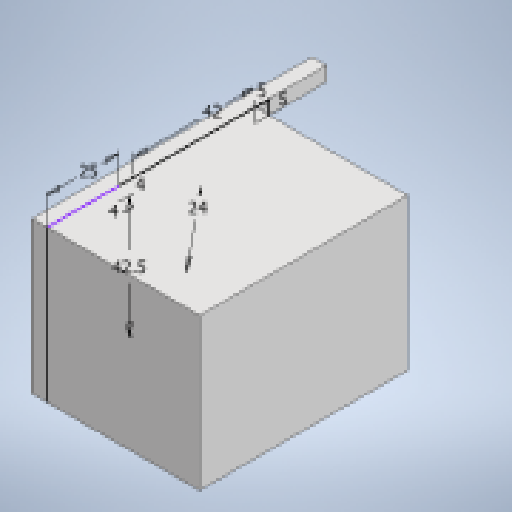
# Autodesk Inventor part: motor_mount
Saved by Autodesk Inventor 2023 (Build 270158000, 158)
## iProperties
Created: 2022-10-01
Part Number: motor_mount
Material: Generic
Document SubType Name: Modeling
Designer: carso
Density: 1 g/cm^3
Appearance: Default
Author: carso
Autodesk Inventor part; units mm, degrees
ref_plane "YZ Plane" through (0, 0, 0) normal (1, 0, 0) x (0, 1, 0)
ref_plane "XZ Plane" through (0, 0, 0) normal (0, 1, 0) x (-1, 0, 0)
ref_plane "XY Plane" through (0, 0, 0) normal (0, 0, 1) x (1, 0, 0)
sketch "Sketch1" plane through (0, 0, 0) normal (1, 0, 0) x (0, 1, 0)
  line L0 (21.25, -21) -> (-21.25, -21)
  line L1 (-21.25, -21) -> (-21.25, 21)
  line L2 (-21.25, 21) -> (21.25, 21)
  line L3 (21.25, 21) -> (21.25, -21)
  line L4 (21.25, -21) -> (-21.25, 21) construction
  line L5 (-21.25, -21) -> (21.25, 21) construction
  line L6 (-26.25, 26) -> (26.25, 26)
  line L7 (26.25, 26) -> (26.25, -26)
  line L8 (26.25, -26) -> (-26.25, -26)
  line L9 (-26.25, -26) -> (-26.25, 26)
  line L10 (-26.25, 26) -> (26.25, -26) construction
  line L11 (26.25, 26) -> (-26.25, -26) construction
  line L12 (17.25, 21) -> (21.25, 17)
  line L13 (-26.25, 0) -> (26.25, 0)
  line L14 (0, 26) -> (0, -26)
  line L15 (21.25, -21) -> (-21.25, 21) construction
  line L16 (-17.25, 21) -> (-21.25, 17)
  line L17 (21.25, -21) -> (26.25, -21)
  line L18 (-21.25, -21) -> (-26.25, -21)
  circle A0 centre (0, 0) radius 12
  line L19 (-26.25, 26) -> (26.25, 26)
  line L20 (26.25, 26) -> (26.25, 51)
  line L21 (26.25, 51) -> (-26.25, 51)
  line L22 (-26.25, 51) -> (-26.25, 26)
  point P0 (-21.25, 17)
  point P1 (-17.25, 21)
  point P2 (-21.25, 0)
  point P3 (-12, 0)
  point P4 (12, 0)
  point P5 (21.25, 0)
  dimension "d0" = 42.5
  dimension "d1" = 42
  dimension "d2" = 5
  dimension "d3" = 5
  dimension "d4" = 4
  dimension "d5" = 4
  dimension "d8" = 24
  dimension "d15" = 25
  constraints: 46 end point, 8 midpoint, 6 parallel, 5 point on line, 4 perpendicular, 3 horizontal, 2 symmetric about line, 1 centre point, 1 coincident
  measures "d0" distance of L1.end L2.end
  measures "d1" distance between parallel lines of L0 L2
  measures "d2" distance between parallel lines of L8 L0
  measures "d3" distance between parallel lines of L7 L3
  measures "d4" distance of L12.end L2.end
  measures "d5" distance of L2.end L12.start
  measures "d8" diameter of A0
  measures "d15" distance between parallel lines of L6 L21
extrude "Extrusion1" add sketch "Sketch1" along normal blind 48 contours L3 L13 L7 L17 | L3 L2 L14 L6 L7 L13 | L18 L9 L13 L1 | L12 L2 L3 | L13 L9 L6 L14 L2 L1 | L6 L22 L21 L20 | L1 L2 L16
extrude "Extrusion2" add sketch "Sketch1" against normal blind 5 contours L3 L13 L7 L17 | L13 A0 L14 L2 L12 L3 | L3 L2 L14 L6 L7 L13 | L18 L9 L13 L1 | L12 L2 L3 | L13 L9 L6 L14 L2 L1 | L1 L16 L2 L14 A0 L13 | L6 L22 L21 L20 | L1 L2 L16
sketch "Sketch2" plane through (48, 0, 0) normal (1, 0, 0) x (0, 0, -1)
  line L0 (21, 26.25) -> (-51, 26.25)
  line L1 (-51, 26.25) -> (-51, -26.25)
  line L2 (-51, -26.25) -> (21, -26.25)
  line L3 (21, -26.25) -> (21, 26.25)
  point P0 (0, 0)
  point P1 (-26, -26.25)
  constraints: 8 end point, 2 parallel, 1 horizontal, 1 perpendicular
extrude "Extrusion3" add sketch "Sketch2" along normal blind 5
sketch "Sketch4" plane through (-5, -26.25, -21) normal (0, 0, -1) x (-1, 0, 0)
  line L0 (0, 52.5) -> (0, 47.5) projected
  line L1 (-5, 47.5) -> (-53, 47.5) projected
  line L2 (0, 52.5) -> (-5, 52.5)
  line L3 (-5, 52.5) -> (-5, 47.5)
  line L4 (-5, 47.5) -> (0, 47.5)
  line L5 (0, 47.5) -> (0, 52.5)
  line L6 (0, 0) -> (0, 52.5) projected
  line L7 (0, 0) -> (-58, 0) projected
  line L8 (0, 4.8747) -> (-5, 4.8747)
  line L9 (-5, 4.8747) -> (-5, 0)
  line L10 (-5, 0) -> (0, 0)
  line L11 (0, 0) -> (0, 4.8747)
  point P0 (-5, 26.25)
  constraints: 16 end point, 4 parallel, 3 point on line, 2 horizontal, 2 perpendicular
extrude "Extrusion5" add sketch "Sketch4" along normal blind 25
body "Solid1"
